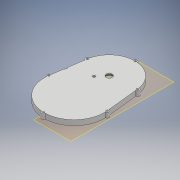
# Autodesk Inventor part: case part 2
Saved by Autodesk Inventor 2017 (Build 210142000, 142)
## iProperties
Created: 2018-04-17
Part Number: case part 2
Material: Generic
Document SubType Name: Modeling
Designer: RKL
Density: 1 g/cm^3
Appearance: Default
Author: RKL
Autodesk Inventor part; units mm, degrees
ref_plane "YZ Plane" through (0, 0, 0) normal (1, 0, 0) x (0, 1, 0)
ref_plane "XZ Plane" through (0, 0, 0) normal (0, 1, 0) x (-1, 0, 0)
ref_plane "XY Plane" through (0, 0, 0) normal (0, 0, 1) x (1, 0, 0)
ref_plane "Work Plane1" through (0, 0, 0) normal (0, 0, 1) x (1, 0, 0)
sketch "Sketch1" plane through (0, 0, 0) normal (0, 0, 1) x (1, 0, 0)
  circle A0 centre (-101.7655, -13.9736) radius 1.397 construction
  circle A1 centre (-129.7655, 19.0264) radius 1.397 construction
  circle A2 centre (-129.7655, -13.9736) radius 1.397 construction
  circle A3 centre (-101.7655, 19.0264) radius 1.397 construction
  circle A4 centre (-43.6844, 106.2389) radius 2.159 projected
  circle A5 centre (-48.0429, -103.7159) radius 2.159 projected
  circle A6 centre (14.7425, 52.5147) radius 2.159 projected
  circle A7 centre (-104.2906, 54.9857) radius 2.159 projected
  arc A8 (-39.1921, 105.9768) -> (-48.1838, 106.1635) centre (-43.6844, 106.2389) ccw projected
  arc A9 (-48.1838, 106.1635) -> (-103.4691, 59.4101) centre (-44.9297, 46.2518) ccw projected
  arc A10 (-103.4691, 59.4101) -> (-104.9457, 50.5336) centre (-104.2906, 54.9857) ccw projected
  line L0 (-104.9457, 50.5336) -> (-109.0664, 22.5264) projected
  line L1 (-133.7655, 22.5264) -> (-109.0664, 22.5264) construction
  line L2 (-133.7655, -17.4736) -> (-133.7655, 22.5264) construction
  line L3 (-133.7655, -17.4736) -> (-119.9083, -25.4741) construction
  arc A11 (-119.9083, -25.4741) -> (-116.3561, -28.0122) centre (-115.8445, -23.5414) ccw projected
  arc A12 (-116.3561, -28.0122) -> (-52.5366, -103.4779) centre (-46.5901, -33.731) ccw projected
  arc A13 (-52.5366, -103.4779) -> (-43.5432, -103.6646) centre (-48.0429, -103.7159) ccw projected
  arc A14 (-43.5432, -103.6646) -> (23.3532, -30.9125) centre (-46.5901, -33.731) ccw projected
  arc A15 (23.3532, -30.9125) -> (22.5578, -21.9488) centre (23.0275, -26.4243) ccw projected
  line L4 (22.5578, -21.9488) -> (15.2122, 48.0393) projected
  arc A16 (15.2122, 48.0393) -> (14.1053, 56.9693) centre (14.7425, 52.5147) ccw projected
  arc A17 (14.1053, 56.9693) -> (-39.1921, 105.9768) centre (-44.9297, 46.2518) ccw projected
  circle A18 centre (-115.8445, -23.5414) radius 2.159 projected
  circle A19 centre (23.0275, -26.4243) radius 2.159 projected
  circle A20 centre (-44.9297, 46.2518) radius 17.5 projected
  circle A21 centre (-46.5901, -33.731) radius 17.5 projected
  circle A22 centre (-112.6295, 11.4221) radius 4 construction
  circle A23 centre (-121.7655, -6.3693) radius 4 construction
  arc A24 (-115.1894, -19.0893) -> (-119.9083, -25.4741) centre (-115.8445, -23.5414) ccw
  line L5 (-109.0664, 22.5264) -> (-115.1894, -19.0893)
  point P0 (0, 0)
  constraints: 2 end point, 2 point on circle, 1 centre point, 1 coincident, 1 collinear
extrude "Extrusion1" add sketch "Sketch1" along normal blind 10
sketch "Sketch2" plane through (0, 0, 10) normal (0, 0, 1) x (1, 0, 0)
  circle A0 centre (-112.6295, 11.4221) radius 4 projected
  point P0 (0, 0)
extrude "Extrusion2" cut sketch "Sketch2" against normal through all
sketch "Sketch3" plane through (0, 0, 10) normal (0, 0, 1) x (1, 0, 0)
  arc A0 (-111.2528, 7.6664) -> (-110.2294, 14.622) centre (-112.6295, 11.4221) ccw projected
  line L0 (-111.2528, 7.6664) -> (-115.1894, -19.0893) projected
  arc A1 (-115.1894, -19.0893) -> (-116.3561, -28.0122) centre (-115.8445, -23.5414) ccw projected
  arc A2 (-116.3561, -28.0122) -> (-52.5366, -103.4779) centre (-46.5901, -33.731) ccw projected
  arc A3 (-52.5366, -103.4779) -> (-43.5432, -103.6646) centre (-48.0429, -103.7159) ccw projected
  arc A4 (-43.5432, -103.6646) -> (23.3532, -30.9125) centre (-46.5901, -33.731) ccw projected
  arc A5 (23.3532, -30.9125) -> (22.5578, -21.9488) centre (23.0275, -26.4243) ccw projected
  line L1 (22.5578, -21.9488) -> (15.2122, 48.0393) projected
  arc A6 (15.2122, 48.0393) -> (14.1053, 56.9693) centre (14.7425, 52.5147) ccw projected
  arc A7 (14.1053, 56.9693) -> (-39.1921, 105.9768) centre (-44.9297, 46.2518) ccw projected
  arc A8 (-39.1921, 105.9768) -> (-48.1838, 106.1635) centre (-43.6844, 106.2389) ccw projected
  arc A9 (-48.1838, 106.1635) -> (-103.4691, 59.4101) centre (-44.9297, 46.2518) ccw projected
  arc A10 (-103.4691, 59.4101) -> (-104.9457, 50.5336) centre (-104.2906, 54.9857) ccw projected
  line L2 (-104.9457, 50.5336) -> (-110.2294, 14.622) projected
  circle A11 centre (-43.6844, 106.2389) radius 2.159 projected
  circle A12 centre (-48.0429, -103.7159) radius 2.159 projected
  circle A13 centre (14.7425, 52.5147) radius 2.159 projected
  circle A14 centre (-104.2906, 54.9857) radius 2.159 projected
  circle A15 centre (-115.8445, -23.5414) radius 2.159 projected
  circle A16 centre (23.0275, -26.4243) radius 2.159 projected
  circle A17 centre (-44.9297, 46.2518) radius 17.5 projected
  circle A18 centre (-46.5901, -33.731) radius 17.5 projected
  circle A19 centre (-46.5901, -33.731) radius 7
  circle A20 centre (-44.9297, 46.2518) radius 7
  point P0 (0, 0)
  dimension "d4" = 14
  constraints: 2 centre point, 2 coincident, 1 equal radius
  measures "d4" diameter of A19
extrude "Extrusion3" add sketch "Sketch3" along normal blind 2 contours A0 L2 A10 A9 A8 A7 A6 L1 A5 A4 A3 A2 A1 L0 | A17 | A18 | A19
sketch "Sketch4" plane through (0, 0, 12) normal (0, 0, 1) x (1, 0, 0)
  circle A0 centre (-61.4531, 27.4907) radius 3 projected
  point P0 (0, 0)
extrude "Extrusion4" cut sketch "Sketch4" against normal through all
sketch "Sketch5" plane through (0, 0, 0) normal (0, 0, -1) x (-1, 0, 0)
  circle A0 centre (61.4531, 27.4907) radius 3 projected
  arc A1 (110.2294, 14.622) -> (111.2528, 7.6664) centre (112.6295, 11.4221) ccw projected
  line L0 (110.2294, 14.622) -> (104.9457, 50.5336) projected
  arc A2 (104.9457, 50.5336) -> (103.4691, 59.4101) centre (104.2906, 54.9857) ccw projected
  arc A3 (103.4691, 59.4101) -> (48.1838, 106.1635) centre (44.9297, 46.2518) ccw projected
  arc A4 (48.1838, 106.1635) -> (39.1921, 105.9768) centre (43.6844, 106.2389) ccw projected
  arc A5 (39.1921, 105.9768) -> (-14.1053, 56.9693) centre (44.9297, 46.2518) ccw projected
  arc A6 (-14.1053, 56.9693) -> (-15.2122, 48.0393) centre (-14.7425, 52.5147) ccw projected
  line L1 (-15.2122, 48.0393) -> (-22.5578, -21.9488) projected
  arc A7 (-22.5578, -21.9488) -> (-23.3532, -30.9125) centre (-23.0275, -26.4243) ccw projected
  arc A8 (-23.3532, -30.9125) -> (43.5432, -103.6646) centre (46.5901, -33.731) ccw projected
  arc A9 (43.5432, -103.6646) -> (52.5366, -103.4779) centre (48.0429, -103.7159) ccw projected
  arc A10 (52.5366, -103.4779) -> (116.3561, -28.0122) centre (46.5901, -33.731) ccw projected
  arc A11 (116.3561, -28.0122) -> (115.1894, -19.0893) centre (115.8445, -23.5414) ccw projected
  line L2 (115.1894, -19.0893) -> (111.2528, 7.6664) projected
  circle A12 centre (46.5901, -33.731) radius 17.5 projected
  circle A13 centre (44.9297, 46.2518) radius 17.5 projected
  circle A14 centre (-23.0275, -26.4243) radius 2.159 projected
  circle A15 centre (115.8445, -23.5414) radius 2.159 projected
  circle A16 centre (104.2906, 54.9857) radius 2.159 projected
  circle A17 centre (-14.7425, 52.5147) radius 2.159 projected
  circle A18 centre (48.0429, -103.7159) radius 2.159 projected
  circle A19 centre (43.6844, 106.2389) radius 2.159 projected
  arc A20 (25.4655, -37.731) -> (42.5901, -54.8556) centre (46.5901, -33.731) ccw
  arc A21 (50.5901, -54.8556) -> (67.7147, -37.731) centre (46.5901, -33.731) ccw
  arc A22 (42.5901, -12.6063) -> (25.4655, -29.731) centre (46.5901, -33.731) ccw
  arc A23 (67.7147, -29.731) -> (50.5901, -12.6063) centre (46.5901, -33.731) ccw
  arc A24 (23.8051, 42.2518) -> (40.9297, 25.1272) centre (44.9297, 46.2518) ccw
  arc A25 (66.0543, 50.2518) -> (48.9297, 67.3764) centre (44.9297, 46.2518) ccw
  arc A26 (40.9297, 67.3764) -> (23.8051, 50.2518) centre (44.9297, 46.2518) ccw
  arc A27 (48.9297, 25.1272) -> (54.4713, 26.9851) centre (44.9297, 46.2518) ccw
  arc A28 (62.8367, 34.3526) -> (66.0543, 42.2518) centre (44.9297, 46.2518) ccw
  arc A29 (54.4713, 26.9851) -> (62.8367, 34.3526) centre (61.4531, 27.4907) ccw
  arc A30 (50.5901, -98.6078) -> (111.4669, -37.731) centre (46.5901, -33.731) ccw
  arc A31 (-18.2867, -37.731) -> (42.5901, -98.6078) centre (46.5901, -33.731) ccw
  arc A32 (40.9297, 101.1062) -> (-9.9246, 50.2518) centre (44.9297, 46.2518) ccw
  arc A33 (99.7841, 50.2518) -> (48.9297, 101.1062) centre (44.9297, 46.2518) ccw
  line L3 (42.5901, -54.8556) -> (42.5901, -98.6078)
  line L4 (-18.2867, -37.731) -> (25.4655, -37.731)
  line L5 (50.5901, -54.8556) -> (50.5901, -98.6078)
  line L6 (111.4669, -37.731) -> (67.7147, -37.731)
  line L7 (67.7147, -29.731) -> (111.7013, -29.731)
  line L8 (111.7013, -29.731) -> (106.9944, 2.2604)
  line L9 (106.9944, 2.2604) -> (50.5901, 2.2604)
  line L10 (50.5901, 2.2604) -> (50.5901, -12.6063)
  arc A34 (52.5366, -103.4779) -> (116.3561, -28.0122) centre (46.5901, -33.731) ccw construction
  line L11 (46.5901, -33.731) -> (44.9297, 46.2518) construction
  line L12 (115.1894, -19.0893) -> (111.2528, 7.6664) construction
  line L13 (25.4655, -29.731) -> (-18.3471, -29.731)
  line L14 (-18.3471, -29.731) -> (-14.9895, 2.2604)
  line L15 (-14.9895, 2.2604) -> (42.5901, 2.2604)
  line L16 (42.5901, 2.2604) -> (42.5901, -12.6063)
  line L17 (-15.2122, 48.0393) -> (-22.5578, -21.9488) projected
  line L18 (48.9297, 25.1272) -> (48.9297, 10.2604)
  line L19 (48.9297, 10.2604) -> (105.8173, 10.2604)
  line L20 (105.8173, 10.2604) -> (101.1104, 42.2518)
  line L21 (101.1104, 42.2518) -> (66.0543, 42.2518)
  line L22 (40.9297, 25.1272) -> (40.9297, 10.2604)
  line L23 (40.9297, 10.2604) -> (-14.1498, 10.2604)
  line L24 (-14.1498, 10.2604) -> (-10.7922, 42.2518)
  line L25 (-10.7922, 42.2518) -> (23.8051, 42.2518)
  line L26 (23.8051, 50.2518) -> (-9.9246, 50.2518)
  line L27 (40.9297, 67.3764) -> (40.9297, 101.1062)
  line L28 (48.9297, 67.3764) -> (48.9297, 101.1062)
  line L29 (66.0543, 50.2518) -> (99.7841, 50.2518)
  point P0 (0, 0)
  point P1 (45.7599, 6.2604)
  dimension "d9" = 4
  dimension "d10" = 4
  dimension "d11" = 4
  dimension "d12" = 4
  dimension "d13" = 5
  dimension "d14" = 5
  dimension "d15" = 4
  dimension "d16" = 4
  dimension "d17" = 4
  dimension "d18" = 4
  dimension "d19" = 5
  dimension "d20" = 4
  dimension "d21" = 4
  dimension "d22" = 4
  dimension "d23" = 4
  dimension "d24" = 5
  dimension "d25" = 4
  dimension "d26" = 4
  dimension "d27" = 4
  dimension "d28" = 4
  dimension "d29" = 4
  dimension "d30" = 5
  dimension "d31" = 4
  dimension "d32" = 4
  dimension "d33" = 5
  dimension "d34" = 5
  dimension "d35" = 4
  dimension "d36" = 4
  dimension "d37" = 5
  dimension "d38" = 4
  dimension "d39" = 4
  dimension "d40" = 4
  dimension "d41" = 4
  dimension "d42" = 4
  dimension "d43" = 4
  constraints: 50 end point, 30 point on circle, 14 centre point, 14 coincident, 8 horizontal, 7 vertical, 6 parallel, 3 perpendicular, 2 concentric, 1 midpoint
  measures "d9" radial gap between concentric circles of A12 A20
  measures "d10" distance from line of A8.centre L3
  measures "d11" distance from line of A30.centre L4
  measures "d12" distance from line of A8.centre L5
  measures "d13" radial gap between concentric circles of A8 A31
  measures "d14" radial gap between concentric circles of A10 A30
  measures "d15" radial gap between concentric circles of A12 A21
  measures "d16" distance from line of A10.centre L6
  measures "d17" radial gap between concentric circles of A12 A23
  measures "d18" distance from line of A10.centre L7
  measures "d19" distance between parallel lines of L2 L8
  measures "d20" distance from line of A8.centre L10
  measures "d21" distance from line of A30.centre L13
  measures "d22" distance from line of A12.centre L16
  measures "d23" distance from line of point (45.76, 6.26) L15
  measures "d24" distance between parallel lines of L1 L14
  measures "d25" radial gap between concentric circles of A0 A29
  measures "d26" radial gap between concentric circles of A13 A27
  measures "d27" radial gap between concentric circles of A13 A28
  measures "d28" distance from line of point (45.76, 6.26) L19
  measures "d29" distance from line of A3.centre L18
  measures "d30" distance between parallel lines of L0 L20
  measures "d31" distance from line of A3.centre L21
  measures "d32" radial gap between concentric circles of A13 A25
  measures "d33" radial gap between concentric circles of A3 A33
  measures "d34" radial gap between concentric circles of A5 A32
  measures "d35" distance from line of A3.centre L22
  measures "d36" distance from line of point (45.76, 6.26) L23
  measures "d37" distance between parallel lines of L1 L24
  measures "d38" distance from line of A3.centre L25
  measures "d39" distance from line of A5.centre L26
  measures "d40" distance from line of A3.centre L27
  measures "d41" distance from line of A3.centre L28
  measures "d42" distance from line of A3.centre L29
  measures "d43" distance from line of point (45.76, 6.26) L9
extrude "Extrusion5" cut sketch "Sketch5" against normal up to surface (10 mm away) contours A20 L3 A31 L4 | A21 L6 A30 L5 | A22 L13 L14 L15 L16 | A23 L10 L9 L8 L7 | A24 L22 L23 L24 L25 | A25 L28 A33 L29 | A26 L26 A32 L27 | A27 A29 A28 L21 L20 L19 L18
body "Solid1"
